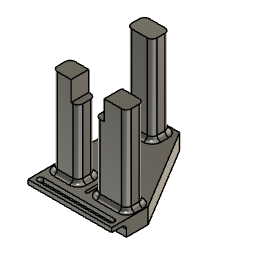
battery_fixture_typeB v7 (Autodesk Fusion 360 design; units mm, degrees)
Autodesk Fusion 360 part; units mm, degrees
sketch "スケッチ1" plane through (0, 0, 0) normal (0, 0, 1) x (1, 0, 0)
  line L0 (0, 0) -> (14, 0)
  line L1 (14, 0) -> (14, 10)
  line L2 (14, 10) -> (0, 10)
  line L3 (0, 10) -> (0, 0)
  line L4 (21.8, 0) -> (38.8, 0)
  line L5 (38.8, 0) -> (38.8, 10)
  line L6 (38.8, 10) -> (21.8, 10)
  line L7 (21.8, 10) -> (21.8, 0)
  line L8 (0.5, 9.5) -> (0.5, 0.5)
  line L9 (0.5, 0.5) -> (13.5, 0.5)
  line L10 (13.5, 0.5) -> (13.5, 9.5)
  line L11 (13.5, 9.5) -> (0.5, 9.5)
  line L12 (22.3, 0.5) -> (38.3, 0.5)
  line L13 (38.3, 0.5) -> (38.3, 9.5)
  line L14 (38.3, 9.5) -> (22.3, 9.5)
  line L15 (22.3, 9.5) -> (22.3, 0.5)
  line L16 (0, 38) -> (14, 38)
  line L17 (14, 38) -> (14, 48)
  line L18 (14, 48) -> (0, 48)
  line L19 (0, 48) -> (0, 38)
  line L20 (0.5, 38.5) -> (13.5, 38.5)
  line L21 (13.5, 38.5) -> (13.5, 47.5)
  line L22 (13.5, 47.5) -> (0.5, 47.5)
  line L23 (0.5, 47.5) -> (0.5, 38.5)
  line L24 (-2, 50) -> (-2, -2)
  line L25 (-2, -2) -> (40.8, -2)
  line L26 (40.8, -2) -> (40.8, 9.0983)
  line L27 (40.8, 9.0983) -> (16, 50)
  line L28 (16, 50) -> (-2, 50)
  line L29 (17.95, 10) -> (19.45, 10)
  line L30 (19.45, 10) -> (19.45, 0)
  line L31 (19.45, 0) -> (17.95, 0)
  line L32 (17.95, 0) -> (17.95, 10)
  line L33 (20.2, 10) -> (20.2, 0)
  line L34 (17.2, 10) -> (17.2, 0)
  arc A0 (19.45, 10) -> (17.95, 10) centre (18.7, 10) ccw
  arc A1 (20.2, 10) -> (17.2, 10) centre (18.7, 10) ccw
  arc A2 (17.95, 0) -> (19.45, 0) centre (18.7, 0) ccw
  arc A3 (17.2, 0) -> (20.2, 0) centre (18.7, 0) ccw
  line L35 (-2, -2) -> (40.8, -2)
  line L36 (40.8, -2) -> (40.8, -6.35)
  line L37 (40.8, -6.35) -> (-2, -6.35)
  line L38 (-2, -6.35) -> (-2, -2)
  line L39 (-2, -6.35) -> (40.8, -6.35)
  line L40 (40.8, -6.35) -> (40.8, -9.55)
  line L41 (40.8, -9.55) -> (-2, -9.55)
  line L42 (-2, -9.55) -> (-2, -6.35)
  circle A4 centre (1.2, -6.35) radius 1.5
  circle A5 centre (37.6, -6.35) radius 1.5
  line L43 (1.2, -4.85) -> (37.6, -4.85)
  line L44 (1.2, -7.85) -> (37.6, -7.85)
  dimension "d1" = 14
  dimension "d2" = 10
  dimension "d3" = 17
  dimension "d4" = 10
  dimension "d5" = 7.8
  dimension "d6" = -0.5
  dimension "d7" = -0.5
  dimension "d8" = 14
  dimension "d9" = 10
  dimension "d10" = 28
  dimension "d11" = -0.5
  dimension "d12" = 2
  dimension "d13" = 2
  dimension "d14" = 2
  dimension "d15" = 14
  dimension "d16" = 2
  dimension "d17" = 2
  dimension "d39" = 3.95
  dimension "d40" = 1.5
  dimension "d41" = 0.75
  dimension "d42" = 0.75
  dimension "d46" = 4.35
  dimension "d47" = 3.2
  dimension "d48" = 3
  dimension "d49" = 3
  dimension "d50" = 3.2
  dimension "d51" = 3.2
  constraint horizontal L0
  constraint vertical L1
  constraint horizontal L2
  constraint vertical L3
  constraint coincident L0.start L3.end
  constraint horizontal L4
  constraint vertical L5
  constraint horizontal L6
  constraint vertical L7
  constraint horizontal L16
  constraint vertical L17
  constraint horizontal L18
  constraint vertical L19
  constraint parallel L23 L24
  constraint perpendicular L24 L25
  constraint perpendicular L12 L26
  constraint perpendicular L24 L28
  constraint horizontal L29
  constraint vertical L30
  constraint horizontal L31
  constraint vertical L32
  constraint perpendicular L29 L33
  constraint perpendicular L31 L34
  constraint midpoint L29 A0.centre
  constraint coincident A0.centre A1.centre
  constraint coincident A2.centre A3.centre
  constraint horizontal L35
  constraint vertical L36
  constraint horizontal L37
  constraint vertical L38
  constraint horizontal L39
  constraint vertical L40
  constraint horizontal L41
  constraint vertical L42
  constraint coincident L39 A4.centre
  constraint coincident L39 A5.centre
  constraint coincident A4 L43.start
  constraint tangent A4 L43
  constraint parallel L37 L43
  constraint coincident A4 L44.start
  constraint coincident A5 L44.end
  constraint tangent A5 L44
  constraint parallel L41 L44
  measures "d1" distance of L1.end L2.end
  measures "d2" distance of L0.end L1.end
  measures "d3" distance of L5.end L6.end
  measures "d4" distance of L4.end L5.end
  measures "d5" distance of L1 L7
  measures "d8" distance of L16.start L16.end
  measures "d9" distance of L16.start L18.end
  measures "d10" distance of L2 L16
  measures "d12" distance of L18 L28
  measures "d13" distance of L19 L24
  measures "d14" distance of L17 L27.end
  measures "d15" distance of L0.start L17
  measures "d16" distance of L0 L25
  measures "d17" distance of L5 L26
  measures "d39" distance of L1 L32
  measures "d40" distance of L30.end L31.end
  measures "d41" distance of L30 L33
  measures "d42" distance of L32 L34
  measures "d46" distance of L24.end L37.end
  measures "d47" distance of L37.end L41.end
  measures "d48" diameter of A4
  measures "d49" diameter of A5
  measures "d50" distance of L42 A4.centre
  measures "d51" distance of L40 A5.centre
extrude "押し出し1" add sketch "スケッチ1" along normal blind 45.2 contours L8 L9 L10 L11 | L12 L13 L14 L15 | L20 L21 L22 L23 makes body 1 at (4.8333, 38.5, 30.1333) makes body 2 at (9.1667, 9.5, 15.0667) makes body 3 at (32.9667, 9.5, 30.1333)
extrude "押し出し2" add sketch "スケッチ1" against normal blind 8 contours L0 L1 L2 L3 | L4 L5 L6 L7 | L8 L9 L10 L11 | L12 L13 L14 L15 | L16 L17 L18 L19 | L20 L21 L22 L23 | L24 L25 L26 L27 L28 L35 | L33 L34 A1 A3 bodies 1 2 3
fillet "フィレット1" radius 2.5 12 edges at (38.3, 9.5, 22.6) (38.3, 0.5, 22.6) (13.5, 9.5, 22.6) (13.5, 0.5, 22.6) (13.5, 38.5, 22.6) (13.5, 47.5, 22.6) (22.3, 0.5, 22.6) (22.3, 9.5, 22.6) (0.5, 38.5, 22.6) (0.5, 47.5, 22.6) (0.5, 9.5, 22.6) (0.5, 0.5, 22.6) on bodies 1
fillet "フィレット2" radius 2 24 edges at (37.5678, 8.7678, 0) (30.3, 9.5, 0) (23.0322, 8.7678, 0) (22.3, 5, 0) (23.0322, 1.2322, 0) (30.3, 0.5, 0) (37.5678, 1.2322, 0) (38.3, 5, 0) (12.7678, 8.7678, 0) (7, 9.5, 0) (1.2322, 8.7678, 0) (0.5, 5, 0) (1.2322, 1.2322, 0) (7, 0.5, 0) (12.7678, 1.2322, 0) (13.5, 5, 0) (12.7678, 46.7678, 0) (7, 47.5, 0) (1.2322, 46.7678, 0) (0.5, 43, 0) (1.2322, 39.2322, 0) (7, 38.5, 0) (12.7678, 39.2322, 0) (13.5, 43, 0) on bodies 1
sketch "スケッチ2" plane through (0, 0.5, 0) normal (0, -1, 0) x (1, 0, 0)
  line L0 (3, 2) -> (11, 2)
  line L1 (11, 2) -> (11, 45.2)
  line L2 (11, 45.2) -> (3, 45.2)
  line L3 (3, 45.2) -> (3, 2)
  line L4 (10, 46) -> (27, 46)
  line L5 (27, 46) -> (27, 35)
  line L6 (27, 35) -> (10, 35)
  line L7 (10, 35) -> (10, 46)
  dimension "d26" = 17
  dimension "d27" = 11
  dimension "d28" = 46
  dimension "d29" = 10
  constraint horizontal L4
  constraint vertical L5
  constraint horizontal L6
  constraint vertical L7
  measures "d26" distance of L4.start L4.end
  measures "d27" distance of L4.end L5.end
  measures "d28" distance of origin L4
  measures "d29" distance of origin L7
extrude "押し出し3" cut sketch "スケッチ2" against normal blind 10 contours L1 L2 L6 L7 | L1 L2 L4 L5 L6 L7 bodies 1
extrude "押し出し5" cut sketch "スケッチ1" against normal blind 9 from surface at -2.2 contours L33 L34 A1 A3 bodies 1
extrude "押し出し6" add sketch "スケッチ1" against normal blind 2.2 contours L25 L35 L36 L37 L38 L39 A4 A5 L43 | L37 L39 L40 L41 L42 A4 A5 L44 bodies 1
fillet "フィレット3" radius 2.2 1 edges at (19.4, -2, -2.2) on bodies 1
